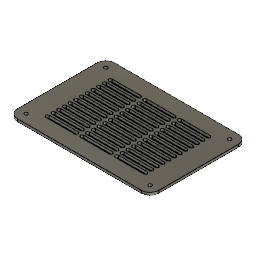
Maker Station v39 (Autodesk Fusion 360 design; units mm, degrees)
Autodesk Fusion 360 part; units mm, degrees
sketch "PiFaceplate" plane through (0, 0, 0) normal (0, 0, 1) x (1, 0, 0)
  line L0 (10, 0) -> (140, 0)
  line L1 (150, 10) -> (150, 100)
  line L2 (140, 110) -> (10, 110)
  line L3 (0, 100) -> (0, 10)
  line L4 (44.2438, 90.3301) -> (105.7438, 90.3301)
  line L5 (107.7438, 88.3301) -> (107.7438, 61.8301)
  line L6 (105.7438, 59.8301) -> (44.2438, 59.8301)
  line L7 (42.2438, 61.8301) -> (42.2438, 88.3301)
  line L8 (20, 40) -> (34.5, 40)
  line L9 (34.5, 40) -> (34.5, 32.75)
  line L10 (34.5, 32.75) -> (20, 32.75)
  line L11 (20, 32.75) -> (20, 40)
  line L12 (34.5, 32.75) -> (20, 32.75)
  line L13 (50, 40) -> (64.5, 40)
  line L14 (64.5, 40) -> (64.5, 32.75)
  line L15 (64.5, 32.75) -> (50, 32.75)
  line L16 (50, 32.75) -> (50, 40)
  line L17 (85.6117, 40) -> (100.1117, 40)
  line L18 (100.1117, 40) -> (100.1117, 32.75)
  line L19 (100.1117, 32.75) -> (85.6117, 32.75)
  line L20 (85.6117, 32.75) -> (85.6117, 40)
  line L21 (115.5147, 40) -> (130.0147, 40)
  line L22 (130.0147, 40) -> (130.0147, 32.75)
  line L23 (130.0147, 32.75) -> (115.5147, 32.75)
  line L24 (115.5147, 32.75) -> (115.5147, 40)
  arc A0 (44.2438, 90.3301) -> (42.2438, 88.3301) centre (44.2438, 88.3301) ccw
  arc A1 (42.2438, 61.8301) -> (44.2438, 59.8301) centre (44.2438, 61.8301) ccw
  arc A2 (107.7438, 88.3301) -> (105.7438, 90.3301) centre (105.7438, 88.3301) ccw
  arc A3 (105.7438, 59.8301) -> (107.7438, 61.8301) centre (105.7438, 61.8301) ccw
  arc A4 (150, 100) -> (140, 110) centre (140, 100) ccw
  arc A5 (140, 0) -> (150, 10) centre (140, 10) ccw
  arc A6 (10, 110) -> (0, 100) centre (10, 100) ccw
  arc A7 (0, 10) -> (10, 0) centre (10, 10) ccw
  line L25 (19.8132, 22.3848) -> (34.3132, 22.3848)
  line L26 (34.3132, 22.3848) -> (34.3132, 15.1348)
  line L27 (34.3132, 15.1348) -> (19.8132, 15.1348)
  line L28 (19.8132, 15.1348) -> (19.8132, 22.3848)
  line L29 (50, 22.3848) -> (64.5, 22.3848)
  line L30 (64.5, 22.3848) -> (64.5, 15.1348)
  line L31 (64.5, 15.1348) -> (50, 15.1348)
  line L32 (50, 15.1348) -> (50, 22.3848)
  line L33 (99.8132, 22.198) -> (85.3132, 22.198)
  line L34 (85.3132, 22.198) -> (85.3132, 14.948)
  line L35 (85.3132, 14.948) -> (99.8132, 14.948)
  line L36 (99.8132, 14.948) -> (99.8132, 22.198)
  line L37 (129.4396, 22.198) -> (114.9396, 22.198)
  line L38 (114.9396, 22.198) -> (114.9396, 14.948)
  line L39 (114.9396, 14.948) -> (129.4396, 14.948)
  line L40 (129.4396, 14.948) -> (129.4396, 22.198)
  circle A8 centre (10, 10) radius 2
  circle A9 centre (140, 10) radius 2
  circle A10 centre (140, 100) radius 2
  circle A11 centre (10, 100) radius 2
  dimension "d1" = 110
  dimension "d2" = 150
  dimension "d3" = 65.5
  dimension "d4" = 30.5
  dimension "d5" = 14.5
  dimension "d6" = 7.25
  dimension "d7" = 14.5
  dimension "d8" = 7.25
  dimension "d9" = 14.5
  dimension "d10" = 7.25
  dimension "d11" = 14.5
  dimension "d12" = 7.25
  dimension "d22" = 2
  dimension "d23" = 2
  dimension "d24" = 2
  dimension "d25" = 2
  dimension "d26" = 10
  dimension "d27" = 10
  dimension "d28" = 10
  dimension "d29" = 10
  dimension "d36" = 14.5
  dimension "d37" = 7.25
  dimension "d38" = 14.5
  dimension "d39" = 7.25
  dimension "d40" = 14.5
  dimension "d41" = 7.25
  dimension "d42" = 14.5
  dimension "d43" = 7.25
  dimension "d44" = 4
  dimension "d45" = 4
  dimension "d46" = 4
  dimension "d47" = 4
  measures "d22" radius of A0
  measures "d23" radius of A1
  measures "d24" radius of A2
  measures "d25" radius of A3
  measures "d26" radius of A4
  measures "d27" radius of A5
  measures "d28" radius of A6
  measures "d29" radius of A7
  measures "d36" distance of origin
  measures "d39" distance of origin
  measures "d41" distance of origin
  measures "d43" distance of origin
  measures "d44" diameter of A8
  measures "d45" diameter of A9
  measures "d46" diameter of A10
  measures "d47" diameter of A11
sketch "PiFaceplateUSB" plane through (0, 30, 0) normal (0, 1, 0) x (-1, 0, 0)
  line L0 (-15, -26) -> (-15, 0)
  line L1 (-135, 0) -> (-135, -26)
  line L2 (-135, -26) -> (-15, -26)
  line L3 (-132.2416, -2.0374) -> (-113.1416, -2.0374)
  line L4 (-113.1416, -2.0374) -> (-113.1416, -16.6374)
  line L5 (-113.1416, -16.6374) -> (-132.2416, -16.6374)
  line L6 (-132.2416, -16.6374) -> (-132.2416, -2.0374)
  line L7 (-102.384, -2.1628) -> (-83.284, -2.1628)
  line L8 (-83.284, -2.1628) -> (-83.284, -16.7628)
  line L9 (-83.284, -16.7628) -> (-102.384, -16.7628)
  line L10 (-102.384, -16.7628) -> (-102.384, -2.1628)
  line L11 (-66.6366, -2.2196) -> (-47.5366, -2.2196)
  line L12 (-47.5366, -2.2196) -> (-47.5366, -16.8196)
  line L13 (-47.5366, -16.8196) -> (-66.6366, -16.8196)
  line L14 (-66.6366, -16.8196) -> (-66.6366, -2.2196)
  line L15 (-37.0103, -2.4202) -> (-17.9103, -2.4202)
  line L16 (-17.9103, -2.4202) -> (-17.9103, -17.0202)
  line L17 (-17.9103, -17.0202) -> (-37.0103, -17.0202)
  line L18 (-37.0103, -17.0202) -> (-37.0103, -2.4202)
  line L19 (-135, 0) -> (-15, 0)
  line L20 (-15, 0) -> (-15, -21)
  line L21 (-20, -26) -> (-130, -26)
  line L22 (-135, -21) -> (-135, 0)
  arc A0 (-135, -21) -> (-130, -26) centre (-130, -21) ccw
  arc A1 (-20, -26) -> (-15, -21) centre (-20, -21) ccw
  line L23 (-15, 0) -> (-135, 0)
  dimension "d55" = 19.1
  dimension "d56" = 14.6
  dimension "d57" = 19.1
  dimension "d58" = 14.6
  dimension "d59" = 19.1
  dimension "d60" = 14.6
  dimension "d61" = 19.1
  dimension "d62" = 14.6
  dimension "d73" = 5
  dimension "d74" = 5
  measures "d73" radius of A0
  measures "d74" radius of A1
combine "Combine1" [no effect]
sketch "SwitchPlate" plane through (0, 0, 0) normal (0, 0, 1) x (1, 0, 0)
  line L0 (-102, 110) -> (-10.6, 110)
  line L1 (-0.6, 100) -> (-0.6, 10)
  line L2 (-10.6, 0) -> (-102, 0)
  line L3 (-112, 10) -> (-112, 100)
  arc A0 (-102, 110) -> (-112, 100) centre (-102, 100) ccw
  arc A1 (-0.6, 100) -> (-10.6, 110) centre (-10.6, 100) ccw
  arc A2 (-112, 10) -> (-102, 0) centre (-102, 10) ccw
  arc A3 (-10.6, 0) -> (-0.6, 10) centre (-10.6, 10) ccw
  circle A4 centre (-102, 100) radius 2
  circle A5 centre (-10.6, 100) radius 2
  circle A6 centre (-10.6, 10) radius 2
  circle A7 centre (-102, 10) radius 2
  circle A8 centre (-79.1, 91.075) radius 8
  circle A9 centre (-55.3, 91.075) radius 8
  circle A10 centre (-31.5, 91.075) radius 8
  circle A11 centre (-79.1, 73.225) radius 8
  circle A12 centre (-55.3, 73.225) radius 8
  circle A13 centre (-31.5, 73.225) radius 8
  circle A14 centre (-79.1, 55.375) radius 8
  circle A15 centre (-55.3, 55.375) radius 8
  circle A16 centre (-31.5, 55.375) radius 8
  circle A17 centre (-79.1, 37.525) radius 8
  circle A18 centre (-55.3, 37.525) radius 8
  circle A19 centre (-31.5, 37.525) radius 8
  circle A20 centre (-79.1, 19.675) radius 8
  circle A21 centre (-55.3, 19.675) radius 8
  circle A22 centre (-31.5, 19.675) radius 8
  dimension "d88" = 111.4
  dimension "d89" = 110
  dimension "d90" = 10
  dimension "d91" = 10
  dimension "d92" = 10
  dimension "d93" = 10
  dimension "d94" = 4
  dimension "d95" = 4
  dimension "d96" = 4
  dimension "d97" = 4
  dimension "d128" = 16
  dimension "d129" = 16
  dimension "d130" = 16
  dimension "d131" = 16
  dimension "d132" = 16
  dimension "d133" = 16
  dimension "d134" = 16
  dimension "d135" = 16
  dimension "d136" = 16
  dimension "d137" = 16
  dimension "d138" = 16
  dimension "d139" = 16
  dimension "d140" = 16
  dimension "d141" = 16
  dimension "d142" = 16
  measures "d90" radius of A0
  measures "d91" radius of A1
  measures "d92" radius of A2
  measures "d93" radius of A3
  measures "d94" diameter of A4
  measures "d95" diameter of A5
  measures "d96" diameter of A6
  measures "d97" diameter of A7
  measures "d128" diameter of A8
  measures "d129" diameter of A9
  measures "d130" diameter of A10
  measures "d131" diameter of A11
  measures "d132" diameter of A12
  measures "d133" diameter of A13
  measures "d134" diameter of A14
  measures "d135" diameter of A15
  measures "d136" diameter of A16
  measures "d137" diameter of A17
  measures "d138" diameter of A18
  measures "d139" diameter of A19
  measures "d140" diameter of A20
  measures "d141" diameter of A21
  measures "d142" diameter of A22
extrude "Extrude9" add sketch "SwitchPlate" along normal blind 3 makes body 1
combine "Combine2" [no effect]
combine "Combine3" [no effect]
combine "Combine4" [no effect]
sketch "SwitchBox" plane through (0, 0, 0) normal (0, 1, 0) x (1, 0, 0)
  line L0 (-10, 0) -> (-102, 0)
  line L1 (-112, 10) -> (-112, 98.329)
  line L2 (-102, 108.329) -> (-10, 108.329)
  line L3 (0, 98.329) -> (0, 10)
  arc A0 (-10, 0) -> (0, 10) centre (-10, 10) ccw
  arc A1 (-112, 10) -> (-102, 0) centre (-102, 10) ccw
  arc A2 (0, 98.329) -> (-10, 108.329) centre (-10, 98.329) ccw
  arc A3 (-102, 108.329) -> (-112, 98.329) centre (-102, 98.329) ccw
  line L4 (-102, 10) -> (-10, 98.329) construction
  line L5 (-10, 10) -> (-102, 98.329) construction
  line L6 (-87, 103.329) -> (-25, 103.329)
  line L7 (-15, 93.329) -> (-15, 15)
  line L8 (-25, 5) -> (-87, 5)
  line L9 (-97, 15) -> (-97, 93.329)
  line L10 (-97, 103.329) -> (-15, 5) construction
  line L11 (-15, 103.329) -> (-97, 5) construction
  arc A4 (-25, 5) -> (-15, 15) centre (-25, 15) ccw
  arc A5 (-97, 15) -> (-87, 5) centre (-87, 15) ccw
  arc A6 (-15, 93.329) -> (-25, 103.329) centre (-25, 93.329) ccw
  arc A7 (-87, 103.329) -> (-97, 93.329) centre (-87, 93.329) ccw
  dimension "d214" = 112
  dimension "d215" = 108.329
  dimension "d216" = 10
  dimension "d217" = 10
  dimension "d218" = 10
  dimension "d219" = 10
  dimension "d220" = 92
  dimension "d221" = 88.329
  dimension "d253" = 82
  dimension "d254" = 98.329
  dimension "d255" = 10
  dimension "d256" = 10
  dimension "d257" = 10
  dimension "d258" = 10
  measures "d216" radius of A0
  measures "d217" radius of A1
  measures "d218" radius of A2
  measures "d219" radius of A3
  measures "d220" distance of origin
  measures "d255" radius of A4
  measures "d256" radius of A5
  measures "d257" radius of A6
  measures "d258" radius of A7
sketch "SwitchBoxFloor" plane through (0, 0, 0) normal (0, 1, 0) x (-1, 0, 0)
  line L0 (87, -103.329) -> (25, -103.329)
  line L1 (15, -93.329) -> (15, -15)
  line L2 (25, -5) -> (87, -5)
  line L3 (97, -15) -> (97, -93.329)
  line L4 (97, -103.329) -> (15, -5) construction
  line L5 (15, -103.329) -> (97, -5) construction
  arc A0 (25, -5) -> (15, -15) centre (25, -15) ccw
  arc A1 (97, -15) -> (87, -5) centre (87, -15) ccw
  arc A2 (15, -93.329) -> (25, -103.329) centre (25, -93.329) ccw
  arc A3 (87, -103.329) -> (97, -93.329) centre (87, -93.329) ccw
  circle A4 centre (90.6, -45.7) radius 4
  circle A5 centre (21.5, -45.7) radius 4
  circle A6 centre (21.5, -95) radius 4
  circle A7 centre (90.6, -95) radius 4
  circle A8 centre (90.6, -45.7) radius 2
  circle A9 centre (21.5, -45.7) radius 2
  circle A10 centre (21.5, -95) radius 2
  circle A11 centre (90.6, -95) radius 2
  dimension "d259" = 82
  dimension "d260" = 98.329
  dimension "d261" = 10
  dimension "d262" = 10
  dimension "d263" = 10
  dimension "d264" = 10
  dimension "d422" = 69.1
  dimension "d423" = 49.3
  dimension "d424" = 8
  dimension "d425" = 8
  dimension "d426" = 8
  dimension "d427" = 8
  dimension "d428" = 4
  dimension "d429" = 4
  dimension "d430" = 4
  dimension "d431" = 4
  measures "d261" radius of A0
  measures "d262" radius of A1
  measures "d263" radius of A2
  measures "d264" radius of A3
  measures "d424" diameter of A4
  measures "d425" diameter of A5
  measures "d426" diameter of A6
  measures "d427" diameter of A7
  measures "d428" diameter of A8
  measures "d429" diameter of A9
  measures "d430" diameter of A10
  measures "d431" diameter of A11
extrude "Extrude18" add sketch "SwitchBox" along normal blind 40 separate body makes body 2
draft "Draft5" angle 10 neutral plane through (-10, 0, 0) pull (0, 0, 1) 1 faces at (-5, 40, -41.1097) on bodies 2
hole "Hole5" at (-102, 57.3381, -98.329) direction (0, -0.984808, -0.173648) diameter 4 depth 4 tip angle 180 bodies 2
hole "Hole6" at (-10, 57.3381, -98.329) direction (0, -0.984808, -0.173648) diameter 4 depth 4 tip angle 180 bodies 2
hole "Hole7" at (-102, 41.7633, -10) direction (0, -0.984808, -0.173648) diameter 4 depth 4 tip angle 180 bodies 2
hole "Hole8" at (-10, 41.7633, -10) direction (0, -0.984808, -0.173648) diameter 4 depth 4 tip angle 180 bodies 2
sketch "BoxJoin" plane through (0, 0, 0) normal (1, 0, 0) x (0, 1, 0)
  line L0 (0, 0) -> (40, 0)
  line L1 (40, 0) -> (40, -108.329)
  line L2 (40, -108.329) -> (0, -108.329)
  line L3 (0, -108.329) -> (0, 0)
  line L4 (40, 0) -> (0, -108.329)
  line L5 (40, -108.329) -> (0, 0)
  line L6 (12.5, -84.1645) -> (27.5, -84.1645)
  line L7 (27.5, -84.1645) -> (27.5, -24.1645)
  line L8 (27.5, -24.1645) -> (12.5, -24.1645)
  line L9 (12.5, -24.1645) -> (12.5, -84.1645)
  line L10 (12.5, -84.1645) -> (27.5, -24.1645) construction
  line L11 (27.5, -84.1645) -> (12.5, -24.1645) construction
  line L12 (20, -54.1645) -> (40, -54.1645)
  circle A0 centre (30, -54.1645) radius 2
  dimension "d281" = 108.329
  dimension "d282" = 40
  dimension "d283" = 15
  dimension "d284" = 60
  dimension "d285" = 4
  measures "d283" distance of L0.start
  measures "d285" diameter of A0
hole "Hole9" at (0, 27.5, -84.1645) at (0, 27.5, -24.1645) at (0, 12.5, -24.1645) at (0, 12.5, -84.1645) direction (-1, 0, 0) diameter 4 depth 30 tip angle 180 bodies 2
hole "Hole10" at (0, 30, -54.1645) direction (-1, 0, 0) diameter 30 depth 30 tip angle 180 bodies 2
extrude "Extrude19" add sketch "SwitchBoxFloor" along normal blind 3 contours L0 L1 L2 L3 A0 A1 A2 A3 | A4 | A5 | A6 | A7 | A8 | A9 | A10 | A11 bodies 2
sketch "PowerBox" plane through (0, 0, 0) normal (0, 1, 0) x (1, 0, 0)
  line L0 (48, 95.25) -> (152, 64.75) construction
  line L1 (152, 95.25) -> (48, 64.75) construction
  circle A0 centre (152, 64.75) radius 4
  circle A1 centre (48, 64.75) radius 4
  circle A2 centre (48, 95.25) radius 4
  circle A3 centre (152, 95.25) radius 4
  circle A4 centre (152, 64.75) radius 2
  circle A5 centre (152, 95.25) radius 2
  circle A6 centre (48, 64.75) radius 2
  circle A7 centre (48, 95.25) radius 2
  line L2 (100, 54.1645) -> (100, 5)
  line L3 (30, 108.329) -> (170, 108.329)
  line L4 (180, 98.329) -> (180, 10)
  line L5 (170, 0) -> (30, 0)
  line L6 (20, 10) -> (20, 98.329)
  arc A8 (170, 0) -> (180, 10) centre (170, 10) ccw
  arc A9 (20, 10) -> (30, 0) centre (30, 10) ccw
  arc A10 (180, 98.329) -> (170, 108.329) centre (170, 98.329) ccw
  arc A11 (30, 108.329) -> (20, 98.329) centre (30, 98.329) ccw
  line L7 (45, 103.329) -> (155, 103.329)
  line L8 (165, 93.329) -> (165, 15)
  line L9 (155, 5) -> (45, 5)
  line L10 (35, 15) -> (35, 93.329)
  line L11 (35, 103.329) -> (165, 5) construction
  line L12 (165, 103.329) -> (35, 5) construction
  arc A12 (155, 5) -> (165, 15) centre (155, 15) ccw
  arc A13 (35, 15) -> (45, 5) centre (45, 15) ccw
  arc A14 (165, 93.329) -> (155, 103.329) centre (155, 93.329) ccw
  arc A15 (45, 103.329) -> (35, 93.329) centre (45, 93.329) ccw
  dimension "d452" = 200
  dimension "d453" = 108.329
  dimension "d470" = 30.5
  dimension "d471" = 104
  dimension "d472" = 8
  dimension "d473" = 8
  dimension "d474" = 8
  dimension "d475" = 8
  dimension "d476" = 4
  dimension "d477" = 4
  dimension "d478" = 4
  dimension "d479" = 4
  dimension "d566" = 10
  dimension "d567" = 10
  dimension "d568" = 10
  dimension "d569" = 10
  dimension "d570" = 130
  dimension "d571" = 98.329
  dimension "d572" = 10
  dimension "d573" = 10
  dimension "d574" = 10
  dimension "d575" = 10
  measures "d472" diameter of A0
  measures "d473" diameter of A1
  measures "d474" diameter of A2
  measures "d475" diameter of A3
  measures "d476" diameter of A4
  measures "d477" diameter of A5
  measures "d478" diameter of A6
  measures "d479" diameter of A7
  measures "d566" radius of A8
  measures "d567" radius of A9
  measures "d568" radius of A10
  measures "d569" radius of A11
  measures "d571" distance of origin
  measures "d572" radius of A12
  measures "d573" radius of A13
  measures "d574" radius of A14
  measures "d575" radius of A15
extrude "Extrude56" add sketch "PowerBox" along normal blind 40 separate body contours L3 L4 L5 L6 A8 A9 A10 A11 makes body 3
extrude "Extrude57" add sketch "PowerBox" along normal blind 3 contours L7 L8 L9 L10 A12 A13 A14 A15 bodies 3
extrude "Extrude58" add sketch "PowerBox" along normal blind 8 contours A1 bodies 3
extrude "Extrude59" add sketch "PowerBox" along normal blind 3 contours A6 bodies 3
extrude "Extrude60" add sketch "PowerBox" along normal blind 3 separate body contours A7 makes body 4
extrude "Extrude61" add sketch "PowerBox" along normal blind 8 contours A2 bodies 3 4
extrude "Extrude62" add sketch "PowerBox" along normal blind 3 separate body contours A5 makes body 5
extrude "Extrude63" add sketch "PowerBox" along normal blind 8 contours A3 bodies 3 5
extrude "Extrude64" add sketch "PowerBox" along normal blind 3 separate body contours A4 makes body 6
extrude "Extrude65" add sketch "PowerBox" along normal blind 8 contours A0 bodies 3 6
draft "Draft9" angle 10 neutral plane through (170, 0, 0) pull (0, 0, 1) 1 faces at (175, 40, -41.1097) on bodies 3
move_body "Move7" bodies 3 to x (1, 0, 0) y (0, 1, 0) z (0, 0, 1) at (-20, 0, 0)
hole "Hole50" at (0, 27.5, -84.1645) at (0, 27.5, -24.1645) at (0, 12.5, -24.1645) at (0, 12.5, -84.1645) direction (1, 0, 0) diameter 4 depth 15 tip angle 180 bodies 3
hole "Hole51" at (0, 30.1179, -54.1346) direction (1, 0, 0) diameter 30 depth 15 tip angle 180 bodies 3
hole "Hole52" at (145, 8.5517, -80.2053) direction (1, 0, 0) diameter 9 depth 15 tip angle 180 bodies 3
move_body "Move8" bodies 3 to x (1, 0, 0) y (0, 1, 0) z (0, 0, 1) at (20, 0, 0)
hole "Hole53" at (170, 57.3381, -98.329) direction (0, -0.984808, -0.173648) diameter 4 depth 4 tip angle 180 bodies 3
hole "Hole54" at (170, 41.7633, -10) direction (0, -0.984808, -0.173648) diameter 4 depth 4 tip angle 180 bodies 3
hole "Hole55" at (30, 41.7633, -10) direction (0, -0.984808, -0.173648) diameter 4 depth 4 tip angle 180 bodies 3
hole "Hole56" at (30, 57.3381, -98.329) direction (0, -0.984808, -0.173648) diameter 4 depth 4 tip angle 180 bodies 3
hole "Hole57" at (35, 27.5, -84.1645) direction (-1, 0, 0) diameter 8 depth 4 tip angle 180 bodies 3
hole "Hole58" at (35, 12.5, -84.1645) direction (-1, 0, 0) diameter 8 depth 4 tip angle 180 bodies 3
hole "Hole59" at (35, 27.5, -24.1645) direction (-1, 0, 0) diameter 8 depth 4 tip angle 180 bodies 3
hole "Hole60" at (35, 12.5, -24.1645) direction (-1, 0, 0) diameter 8 depth 4 tip angle 180 bodies 3
sketch "PowerBoxFacePlateWithPiZero" plane through (0, 0, 0) normal (0, 0, 1) x (1, 0, 0)
  line L0 (20, 0) -> (160, 0)
  line L1 (170, 10) -> (170, 100)
  line L2 (160, 110) -> (20, 110)
  line L3 (10, 100) -> (10, 10)
  arc A0 (10, 10) -> (20, 0) centre (20, 10) ccw
  arc A1 (160, 0) -> (170, 10) centre (160, 10) ccw
  arc A2 (20, 110) -> (10, 100) centre (20, 100) ccw
  arc A3 (170, 100) -> (160, 110) centre (160, 100) ccw
  circle A4 centre (20, 10) radius 2
  circle A5 centre (160, 10) radius 2
  circle A6 centre (160, 100) radius 2
  circle A7 centre (20, 100) radius 2
  circle A8 centre (50, 80) radius 6
  circle A9 centre (130, 80) radius 6
  line L4 (120.9659, 48.9991) -> (59.4659, 48.9991)
  line L5 (57.4659, 46.9991) -> (57.4659, 20.4991)
  line L6 (59.4659, 18.4991) -> (120.9659, 18.4991)
  line L7 (122.9659, 20.4991) -> (122.9659, 46.9991)
  line L8 (122.9659, 48.9991) -> (57.4659, 18.4991) construction
  line L9 (57.4659, 48.9991) -> (122.9659, 18.4991) construction
  arc A10 (57.4659, 20.4991) -> (59.4659, 18.4991) centre (59.4659, 20.4991) ccw
  arc A11 (59.4659, 48.9991) -> (57.4659, 46.9991) centre (59.4659, 46.9991) ccw
  arc A12 (120.9659, 18.4991) -> (122.9659, 20.4991) centre (120.9659, 20.4991) ccw
  arc A13 (122.9659, 46.9991) -> (120.9659, 48.9991) centre (120.9659, 46.9991) ccw
  dimension "d631" = 110
  dimension "d632" = 160
  dimension "d633" = 10
  dimension "d634" = 10
  dimension "d635" = 10
  dimension "d636" = 10
  dimension "d637" = 4
  dimension "d638" = 4
  dimension "d639" = 4
  dimension "d640" = 4
  dimension "d641" = 12
  dimension "d642" = 12
  dimension "d643" = 30.5
  dimension "d644" = 65.5
  dimension "d645" = 2
  dimension "d646" = 2
  dimension "d647" = 2
  dimension "d648" = 2
  measures "d632" distance of origin
  measures "d633" radius of A0
  measures "d634" radius of A1
  measures "d635" radius of A2
  measures "d636" radius of A3
  measures "d637" diameter of A4
  measures "d638" diameter of A5
  measures "d639" diameter of A6
  measures "d640" diameter of A7
  measures "d641" diameter of A8
  measures "d642" diameter of A9
  measures "d643" distance of origin
  measures "d645" radius of A10
  measures "d646" radius of A11
  measures "d647" radius of A12
  measures "d648" radius of A13
extrude "Extrude66" add sketch "PowerBoxFacePlateWithPiZero" along normal blind 3 separate body makes body 7
sketch "SmallBoxUsbPlate" plane through (0, 0, 0) normal (0, 0, 1) x (1, 0, 0)
  line L0 (10, 0) -> (101.4, 0)
  line L1 (111.4, 10) -> (111.4, 100)
  line L2 (101.4, 110) -> (10, 110)
  line L3 (0, 100) -> (0, 10)
  arc A0 (0, 10) -> (10, 0) centre (10, 10) ccw
  arc A1 (101.4, 0) -> (111.4, 10) centre (101.4, 10) ccw
  arc A2 (111.4, 100) -> (101.4, 110) centre (101.4, 100) ccw
  arc A3 (10, 110) -> (0, 100) centre (10, 100) ccw
  line L4 (45.45, 22.125) -> (30.95, 22.125)
  line L5 (30.95, 22.125) -> (30.95, 14.875)
  line L6 (30.95, 14.875) -> (45.45, 14.875)
  line L7 (45.45, 14.875) -> (45.45, 22.125)
  line L8 (45.45, 22.125) -> (30.95, 14.875) construction
  line L9 (30.95, 22.125) -> (45.45, 14.875) construction
  line L10 (80.45, 22.125) -> (65.95, 22.125)
  line L11 (65.95, 22.125) -> (65.95, 14.875)
  line L12 (65.95, 14.875) -> (80.45, 14.875)
  line L13 (80.45, 14.875) -> (80.45, 22.125)
  line L14 (80.45, 22.125) -> (65.95, 14.875) construction
  line L15 (65.95, 22.125) -> (80.45, 14.875) construction
  line L16 (45.45, 40.125) -> (30.95, 40.125)
  line L17 (30.95, 40.125) -> (30.95, 32.875)
  line L18 (30.95, 32.875) -> (45.45, 32.875)
  line L19 (45.45, 32.875) -> (45.45, 40.125)
  line L20 (45.45, 40.125) -> (30.95, 32.875) construction
  line L21 (30.95, 40.125) -> (45.45, 32.875) construction
  line L22 (80.45, 40.125) -> (65.95, 40.125)
  line L23 (65.95, 40.125) -> (65.95, 32.875)
  line L24 (65.95, 32.875) -> (80.45, 32.875)
  line L25 (80.45, 32.875) -> (80.45, 40.125)
  line L26 (80.45, 40.125) -> (65.95, 32.875) construction
  line L27 (65.95, 40.125) -> (80.45, 32.875) construction
  line L28 (45.45, 77.125) -> (30.95, 77.125)
  line L29 (30.95, 77.125) -> (30.95, 69.875)
  line L30 (30.95, 69.875) -> (45.45, 69.875)
  line L31 (45.45, 69.875) -> (45.45, 77.125)
  line L32 (45.45, 77.125) -> (30.95, 69.875) construction
  line L33 (30.95, 77.125) -> (45.45, 69.875) construction
  line L34 (80.45, 77.125) -> (65.95, 77.125)
  line L35 (65.95, 77.125) -> (65.95, 69.875)
  line L36 (65.95, 69.875) -> (80.45, 69.875)
  line L37 (80.45, 69.875) -> (80.45, 77.125)
  line L38 (80.45, 77.125) -> (65.95, 69.875) construction
  line L39 (65.95, 77.125) -> (80.45, 69.875) construction
  line L40 (45.45, 95.125) -> (30.95, 95.125)
  line L41 (30.95, 95.125) -> (30.95, 87.875)
  line L42 (30.95, 87.875) -> (45.45, 87.875)
  line L43 (45.45, 87.875) -> (45.45, 95.125)
  line L44 (45.45, 95.125) -> (30.95, 87.875) construction
  line L45 (30.95, 95.125) -> (45.45, 87.875) construction
  line L46 (80.45, 95.125) -> (65.95, 95.125)
  line L47 (65.95, 95.125) -> (65.95, 87.875)
  line L48 (65.95, 87.875) -> (80.45, 87.875)
  line L49 (80.45, 87.875) -> (80.45, 95.125)
  line L50 (80.45, 95.125) -> (65.95, 87.875) construction
  line L51 (65.95, 95.125) -> (80.45, 87.875) construction
  line L52 (94.7, 83.5) -> (16.7, 83.5)
  line L53 (16.7, 83.5) -> (16.7, 81.5)
  line L54 (16.7, 81.5) -> (94.7, 81.5)
  line L55 (94.7, 81.5) -> (94.7, 83.5)
  line L56 (94.7, 83.5) -> (16.7, 81.5) construction
  line L57 (16.7, 83.5) -> (94.7, 81.5) construction
  line L58 (94.7, 28.5) -> (16.7, 28.5)
  line L59 (16.7, 28.5) -> (16.7, 26.5)
  line L60 (16.7, 26.5) -> (94.7, 26.5)
  line L61 (94.7, 26.5) -> (94.7, 28.5)
  line L62 (94.7, 28.5) -> (16.7, 26.5) construction
  line L63 (16.7, 28.5) -> (94.7, 26.5) construction
  circle A4 centre (10, 10) radius 2
  circle A5 centre (10, 100) radius 2
  circle A6 centre (101.4, 100) radius 2
  circle A7 centre (101.4, 10) radius 2
  dimension "d651" = 111.4
  dimension "d652" = 110
  dimension "d653" = 10
  dimension "d654" = 10
  dimension "d655" = 10
  dimension "d656" = 10
  dimension "d661" = 14.5
  dimension "d662" = 7.25
  dimension "d663" = 14.5
  dimension "d664" = 7.25
  dimension "d665" = 14.5
  dimension "d666" = 7.25
  dimension "d667" = 14.5
  dimension "d668" = 7.25
  dimension "d669" = 14.5
  dimension "d670" = 7.25
  dimension "d671" = 7.25
  dimension "d672" = 14.5
  dimension "d673" = 7.25
  dimension "d674" = 14.5
  dimension "d676" = 7.25
  dimension "d677" = 78
  dimension "d678" = 2
  dimension "d679" = 78
  dimension "d680" = 2
  dimension "d687" = 4
  dimension "d688" = 4
  dimension "d689" = 4
  dimension "d690" = 4
  measures "d653" radius of A0
  measures "d654" radius of A1
  measures "d655" radius of A2
  measures "d656" radius of A3
  measures "d662" distance of origin
  measures "d664" distance of origin
  measures "d677" distance of origin
  measures "d679" distance of origin
  measures "d687" diameter of A4
  measures "d688" diameter of A5
  measures "d689" diameter of A6
  measures "d690" diameter of A7
extrude "Extrude73" add sketch "SmallBoxUsbPlate" along normal blind 3 separate body makes body 8
sketch "SmallBoxUsbPlateUsbSupport" plane through (0, 0, 0) normal (0, 1, 0) x (1, 0, 0)
  line L0 (89.7, -24) -> (21.7, -24)
  line L1 (16.7, -19) -> (16.7, 0)
  line L2 (16.7, 0) -> (94.7, 0)
  line L3 (94.7, 0) -> (94.7, -19)
  arc A0 (89.7, -24) -> (94.7, -19) centre (89.7, -19) ccw
  arc A1 (16.7, -19) -> (21.7, -24) centre (21.7, -19) ccw
  circle A2 centre (28.2, -20.35) radius 1.65
  circle A3 centre (28.2, -5.65) radius 1.65
  circle A4 centre (48.2, -20.35) radius 1.65
  circle A5 centre (48.2, -5.65) radius 1.65
  circle A6 centre (63.2, -20.35) radius 1.65
  circle A7 centre (83.2, -20.35) radius 1.65
  circle A8 centre (83.2, -5.65) radius 1.65
  circle A9 centre (63.2, -5.65) radius 1.65
  dimension "d707" = 5
  dimension "d708" = 5
  dimension "d713" = 3.3
  dimension "d714" = 3.3
  dimension "d715" = 3.3
  dimension "d716" = 3.3
  dimension "d717" = 3.3
  dimension "d718" = 3.3
  dimension "d719" = 3.3
  dimension "d720" = 3.3
  measures "d707" radius of A0
  measures "d708" radius of A1
  measures "d713" diameter of A2
  measures "d714" diameter of A3
  measures "d715" diameter of A4
  measures "d716" diameter of A5
  measures "d717" diameter of A6
  measures "d718" diameter of A7
  measures "d719" diameter of A8
  measures "d720" diameter of A9
extrude "Extrude76" add sketch "SmallBoxUsbPlateUsbSupport" along normal blind 2 from surface at 26.5 bodies 8
extrude "Extrude77" add sketch "SmallBoxUsbPlateUsbSupport" along normal blind 2 from surface at 81.5 bodies 8
sketch "ComputeBox" plane through (0, 0, 0) normal (0, 1, 0) x (1, 0, 0)
  arc A0 (155, 5) -> (165, 15) centre (155, 15) ccw
  line L0 (165, 93.329) -> (165, 15)
  line L1 (121.0013, 97.1895) -> (63.0013, 48.1895) construction
  line L2 (155, 5) -> (45, 5)
  line L3 (165, 103.329) -> (35, 5) construction
  line L4 (35, 103.329) -> (165, 5) construction
  line L5 (180, 98.329) -> (180, 10)
  line L6 (35, 15) -> (35, 93.329)
  arc A1 (170, 0) -> (180, 10) centre (170, 10) ccw
  arc A2 (45, 103.329) -> (35, 93.329) centre (45, 93.329) ccw
  circle A3 centre (121.0013, 97.1895) radius 4
  circle A4 centre (63.0013, 48.1895) radius 4
  circle A5 centre (121.0013, 48.1895) radius 4
  arc A6 (20, 10) -> (30, 0) centre (30, 10) ccw
  arc A7 (30, 108.329) -> (20, 98.329) centre (30, 98.329) ccw
  circle A8 centre (63.0013, 97.1895) radius 2
  arc A9 (165, 93.329) -> (155, 103.329) centre (155, 93.329) ccw
  circle A10 centre (121.0013, 97.1895) radius 2
  arc A11 (35, 15) -> (45, 5) centre (45, 15) ccw
  circle A12 centre (121.0013, 48.1895) radius 2
  arc A13 (180, 98.329) -> (170, 108.329) centre (170, 98.329) ccw
  circle A14 centre (63.0013, 97.1895) radius 4
  circle A15 centre (63.0013, 48.1895) radius 2
  line L7 (20, 10) -> (20, 98.329)
  line L8 (63.0013, 97.1895) -> (121.0013, 48.1895) construction
  line L9 (45, 103.329) -> (155, 103.329)
  line L10 (30, 108.329) -> (170, 108.329)
  line L11 (170, 0) -> (30, 0)
  circle A16 centre (170, 10) radius 2
  circle A17 centre (170, 98.329) radius 2
  circle A18 centre (30, 10) radius 2
  circle A19 centre (30, 98.329) radius 2
  dimension "d727" = 200
  dimension "d728" = 108.329
  dimension "d731" = 8
  dimension "d732" = 8
  dimension "d733" = 8
  dimension "d734" = 8
  dimension "d735" = 4
  dimension "d736" = 4
  dimension "d737" = 4
  dimension "d738" = 4
  dimension "d739" = 10
  dimension "d740" = 10
  dimension "d741" = 10
  dimension "d742" = 10
  dimension "d743" = 130
  dimension "d744" = 98.329
  dimension "d745" = 10
  dimension "d746" = 10
  dimension "d747" = 10
  dimension "d748" = 10
  dimension "d805" = 4
  dimension "d806" = 4
  dimension "d807" = 4
  dimension "d808" = 4
  measures "d731" diameter of A5
  measures "d732" diameter of A4
  measures "d733" diameter of A14
  measures "d734" diameter of A3
  measures "d735" diameter of A12
  measures "d736" diameter of A10
  measures "d737" diameter of A15
  measures "d738" diameter of A8
  measures "d739" radius of A1
  measures "d740" radius of A6
  measures "d741" radius of A13
  measures "d742" radius of A7
  measures "d744" distance of origin
  measures "d745" radius of A0
  measures "d746" radius of A11
  measures "d747" radius of A9
  measures "d748" radius of A2
  measures "d805" diameter of A16
  measures "d806" diameter of A17
  measures "d807" diameter of A18
  measures "d808" diameter of A19
extrude "Extrude78" add sketch "ComputeBox" along normal blind 40 separate body contours L5 A1 A6 A7 A13 L7 L10 L11 | A16 | A17 | A18 | A19 makes body 9
extrude "Extrude79" add sketch "ComputeBox" along normal blind 3 contours A0 L0 L2 L6 A2 A9 A11 L9 bodies 9
extrude "Extrude80" add sketch "ComputeBox" along normal blind 3 separate body contours A15 makes body 10
extrude "Extrude81" add sketch "ComputeBox" along normal blind 8 contours A4 bodies 9 10
extrude "Extrude82" add sketch "ComputeBox" along normal blind 3 separate body contours A12 makes body 11
extrude "Extrude83" add sketch "ComputeBox" along normal blind 8 contours A5 bodies 9 11
extrude "Extrude84" add sketch "ComputeBox" along normal blind 3 separate body contours A10 makes body 12
extrude "Extrude85" add sketch "ComputeBox" along normal blind 8 contours A3 bodies 9 12
extrude "Extrude86" add sketch "ComputeBox" along normal blind 8 contours A14 bodies 9
extrude "Extrude87" add sketch "ComputeBox" along normal blind 3 contours A8 bodies 9
draft "Draft10" angle 10 neutral plane through (170, 0, 0) pull (0, 0, 1) 1 faces at (175, 40, -41.1097) on bodies 9
hole "Hole61" at (0, 30, -54.1645) direction (1, 0, 0) diameter 30 depth 200 tip angle 180 bodies 9
hole "Hole62" at (0, 27.5, -24.1645) at (0, 12.5, -24.1645) at (0, 27.5, -84.1645) at (0, 12.5, -84.1645) direction (1, 0, 0) diameter 4 depth 200 tip angle 180 bodies 9
hole "Hole63" at (165, 27.5, -24.1645) direction (1, 0, 0) diameter 8 depth 4 tip angle 180 bodies 9
hole "Hole64" at (165, 12.5, -24.1645) direction (1, 0, 0) diameter 8 depth 4 tip angle 180 bodies 9
hole "Hole65" at (165, 27.5, -84.1645) direction (1, 0, 0) diameter 8 depth 4 tip angle 180 bodies 9
hole "Hole66" at (165, 12.5, -84.1645) direction (1, 0, 0) diameter 8 depth 4 tip angle 180 bodies 9
hole "Hole67" at (35, 27.5, -84.1645) direction (-1, 0, 0) diameter 8 depth 4 tip angle 180 bodies 9
hole "Hole68" at (35, 12.5, -84.1645) direction (-1, 0, 0) diameter 8 depth 4 tip angle 180 bodies 9
hole "Hole69" at (35, 27.5, -24.1645) direction (-1, 0, 0) diameter 8 depth 4 tip angle 180 bodies 9
hole "Hole70" at (35, 12.5, -24.1645) direction (-1, 0, 0) diameter 8 depth 4 tip angle 180 bodies 9
hole "Hole71" at (170, 41.7633, -10) direction (0, -0.984808, -0.173648) diameter 4 depth 4 tip angle 180 bodies 9
hole "Hole72" at (170, 57.3381, -98.329) direction (0, -0.984808, -0.173648) diameter 4 depth 4 tip angle 180 bodies 9
hole "Hole73" at (30, 57.3381, -98.329) direction (0, -0.984808, -0.173648) diameter 4 depth 4 tip angle 180 bodies 9
hole "Hole74" at (30, 41.7633, -10) direction (0, -0.984808, -0.173648) diameter 4 depth 4 tip angle 180 bodies 9
sketch "Sketch33" plane through (0, 0, 0) normal (0, 0, 1) x (1, 0, 0)
  line L0 (10, 0) -> (150, 0)
  line L1 (160, 10) -> (160, 100)
  line L2 (150, 110) -> (10, 110)
  line L3 (0, 100) -> (0, 10)
  arc A0 (0, 10) -> (10, 0) centre (10, 10) ccw
  arc A1 (150, 0) -> (160, 10) centre (150, 10) ccw
  arc A2 (10, 110) -> (0, 100) centre (10, 100) ccw
  arc A3 (160, 100) -> (150, 110) centre (150, 100) ccw
  line L4 (10, 10) -> (150, 100)
  line L5 (150, 10) -> (10, 100)
  dimension "d821" = 160
  dimension "d822" = 110
  dimension "d823" = 10
  dimension "d824" = 10
  dimension "d825" = 10
  dimension "d826" = 10
  measures "d823" radius of A0
  measures "d824" radius of A1
  measures "d825" radius of A2
  measures "d826" radius of A3
extrude "Extrude88" add sketch "Sketch33" along normal blind 3 separate body makes body 13
sketch "Sketch34" plane through (0, 0, 0) normal (0, 0, -1) x (-1, 0, 0)
  arc A0 (-150, 110) -> (-160, 100) centre (-150, 100) ccw construction
  line L0 (-160, 100) -> (-160, 10) construction
  arc A1 (-160, 10) -> (-150, 0) centre (-150, 10) ccw construction
  line L1 (-150, 0) -> (-10, 0) construction
  arc A2 (-10, 0) -> (0, 10) centre (-10, 10) ccw construction
  line L2 (0, 10) -> (0, 100) construction
  arc A3 (0, 100) -> (-10, 110) centre (-10, 100) ccw construction
  line L3 (-10, 110) -> (-150, 110) construction
  line L4 (-102.8467, 21.455) -> (-135.46, 21.455)
  line L5 (-137.46, 19.455) -> (-137.46, 19.54)
  line L6 (-135.46, 17.54) -> (-102.8467, 17.54)
  line L7 (-100.8467, 19.54) -> (-100.8467, 19.455)
  arc A4 (-135.46, 21.455) -> (-137.46, 19.455) centre (-135.46, 19.455) ccw
  arc A5 (-137.46, 19.54) -> (-135.46, 17.54) centre (-135.46, 19.54) ccw
  arc A6 (-102.8467, 17.54) -> (-100.8467, 19.54) centre (-102.8467, 19.54) ccw
  arc A7 (-100.8467, 19.455) -> (-102.8467, 21.455) centre (-102.8467, 19.455) ccw
extrude "Extrude89" add sketch "Sketch34" against normal up to surface (3 mm away) separate body makes body 14
copy_body "CopyPasteBodies2" bodies 14 makes body 15
move_body "MoveBody1" bodies 15 to x (1, 0, 0) y (0, 1, 0) z (0, 0, 1) at (-39.1533, 0, 0)
copy_body "CopyPasteBodies3" bodies 14 makes body 16
move_body "MoveBody2" bodies 16 to x (1, 0, 0) y (0, 1, 0) z (0, 0, 1) at (-78.3067, 0, 0)
copy_body "CopyPasteBodies4" bodies 14 makes body 17
copy_body "CopyPasteBodies5" bodies 15 makes body 18
copy_body "CopyPasteBodies6" bodies 16 makes body 19
move_body "MoveBody3" bodies 17 18 19 to x (1, 0, 0) y (0, 1, 0) z (0, 0, 1) at (0, 6.455, 0)
copy_body "CopyPasteBodies7" bodies 14 makes body 20
copy_body "CopyPasteBodies8" bodies 15 makes body 21
copy_body "CopyPasteBodies9" bodies 16 makes body 22
move_body "MoveBody4" bodies 20 21 22 to x (1, 0, 0) y (0, 1, 0) z (0, 0, 1) at (0, 12.91, 0)
copy_body "CopyPasteBodies10" bodies 14 makes body 23
copy_body "CopyPasteBodies11" bodies 15 makes body 24
copy_body "CopyPasteBodies12" bodies 16 makes body 25
move_body "MoveBody5" bodies 23 24 25 to x (1, 0, 0) y (0, 1, 0) z (0, 0, 1) at (0, 19.365, 0)
copy_body "CopyPasteBodies13" bodies 14 makes body 26
copy_body "CopyPasteBodies14" bodies 15 makes body 27
copy_body "CopyPasteBodies15" bodies 16 makes body 28
move_body "MoveBody6" bodies 26 27 28 to x (1, 0, 0) y (0, 1, 0) z (0, 0, 1) at (0, 25.82, 0)
copy_body "CopyPasteBodies16" bodies 14 makes body 29
copy_body "CopyPasteBodies17" bodies 15 makes body 30
copy_body "CopyPasteBodies18" bodies 16 makes body 31
move_body "MoveBody7" bodies 29 30 31 to x (1, 0, 0) y (0, 1, 0) z (0, 0, 1) at (0, 32.275, 0)
copy_body "CopyPasteBodies19" bodies 14 makes body 32
copy_body "CopyPasteBodies20" bodies 15 makes body 33
copy_body "CopyPasteBodies21" bodies 16 makes body 34
move_body "MoveBody8" bodies 32 33 34 to x (1, 0, 0) y (0, 1, 0) z (0, 0, 1) at (0, 38.73, 0)
copy_body "CopyPasteBodies22" bodies 14 makes body 35
copy_body "CopyPasteBodies23" bodies 15 makes body 36
copy_body "CopyPasteBodies24" bodies 16 makes body 37
move_body "MoveBody9" bodies 35 36 37 to x (1, 0, 0) y (0, 1, 0) z (0, 0, 1) at (0, 45.185, 0)
copy_body "CopyPasteBodies25" bodies 14 makes body 38
copy_body "CopyPasteBodies26" bodies 15 makes body 39
copy_body "CopyPasteBodies27" bodies 16 makes body 40
move_body "MoveBody10" bodies 38 39 40 to x (1, 0, 0) y (0, 1, 0) z (0, 0, 1) at (0, 51.64, 0)
copy_body "CopyPasteBodies28" bodies 14 makes body 41
copy_body "CopyPasteBodies29" bodies 15 makes body 42
copy_body "CopyPasteBodies30" bodies 16 makes body 43
move_body "MoveBody11" bodies 41 42 43 to x (1, 0, 0) y (0, 1, 0) z (0, 0, 1) at (0, 58.095, 0)
copy_body "CopyPasteBodies31" bodies 14 makes body 44
copy_body "CopyPasteBodies32" bodies 15 makes body 45
copy_body "CopyPasteBodies33" bodies 16 makes body 46
move_body "MoveBody12" bodies 44 45 46 to x (1, 0, 0) y (0, 1, 0) z (0, 0, 1) at (0, 64.55, 0)
copy_body "CopyPasteBodies34" bodies 14 makes body 47
copy_body "CopyPasteBodies35" bodies 15 makes body 48
copy_body "CopyPasteBodies36" bodies 16 makes body 49
move_body "MoveBody13" bodies 47 48 49 to x (1, 0, 0) y (0, 1, 0) z (0, 0, 1) at (0, 71.005, 0)
combine "Combine14" operation cut target body 13 tool bodies 14 15 16 17 18 19 20 21 22 23 24 25 26 27 28 29 30 31 32 33 34 35 36 37 38 39 40 41 42 43 44 45 46 47 48 49
hole "Hole75" at (10, 100, 0) at (150, 100, 0) at (150, 10, 0) at (10, 10, 0) direction (0, 0, 1) diameter 4 depth 3 tip angle 180 bodies 13
extrude "Extrude70" [suppressed]
combine "Combine13" [suppressed]
extrude "Extrude71" [suppressed]
extrude "Extrude72" [suppressed]
extrude "Extrude37" [suppressed]
extrude "Extrude35" [suppressed]
extrude "Extrude38" [suppressed]
extrude "Extrude39" [suppressed]
extrude "Extrude40" [suppressed]
extrude "Extrude41" [suppressed]
extrude "Extrude42" [suppressed]
extrude "Extrude43" [suppressed]
extrude "Extrude44" [suppressed]
extrude "Extrude45" [suppressed]
combine "Combine12" [suppressed]
draft "Draft7" [suppressed]
hole "Hole36" [suppressed]
hole "Hole37" [suppressed]
hole "Hole38" [suppressed]
hole "Hole39" [suppressed]
hole "Hole40" [suppressed]
hole "Hole41" [suppressed]
hole "Hole42" [suppressed]
combine "Combine5" [suppressed]
combine "Combine7" [suppressed]
combine "Combine8" [suppressed]
combine "Combine9" [suppressed]
combine "Combine10" [suppressed]
extrude "Extrude28" [suppressed]
extrude "Extrude29" [suppressed]
hole "Hole20" [suppressed]
moveface "MoveFace8" [suppressed]
move_face "OffsetFaces1" [suppressed]
extrude "Extrude30" [suppressed]
hole "Hole21" [suppressed]
move_face "OffsetFaces2" [suppressed]
copy_body "CopyPasteBodies1" [suppressed]
move_body "Move6" [suppressed]
hole "Hole22" [suppressed]
hole "Hole23" [suppressed]
hole "Hole24" [suppressed]
hole "Hole25" [suppressed]
hole "Hole26" [suppressed]
hole "Hole27" [suppressed]
hole "Hole28" [suppressed]
hole "Hole29" [suppressed]
hole "Hole30" [suppressed]
hole "Hole31" [suppressed]
delete_face "DeleteFace2" [suppressed]
delete_face "DeleteFace3" [suppressed]
delete_face "DeleteFace4" [suppressed]
delete_face "DeleteFace5" [suppressed]
extrude "Extrude31" [suppressed]
extrude "Extrude32" [suppressed]
extrude "Extrude33" [suppressed]
extrude "Extrude34" [suppressed]
combine "Combine11" [suppressed]
hole "Hole32" [suppressed]
hole "Hole33" [suppressed]
hole "Hole34" [suppressed]
hole "Hole35" [suppressed]
extrude "Extrude36" [suppressed]
sketch "BoxJoins" plane through (0, 0, 0) normal (1, 0, 0) x (0, 1, 0)
  line L0 (0, 0) -> (25, 0)
  line L1 (25, 0) -> (25, -108.329)
  line L2 (25, -108.329) -> (0, -108.329)
  line L3 (0, -108.329) -> (0, 0)
  circle A0 centre (7.5, -25) radius 2
  circle A1 centre (17.5, -25) radius 2
  circle A2 centre (7.5, -83.329) radius 2
  circle A3 centre (17.5, -83.329) radius 2
  circle A4 centre (18.8333, -54.1645) radius 12.5
  dimension "d236" = 108.329
  dimension "d237" = 25
  dimension "d238" = 58.329
  dimension "d239" = 10
  dimension "d240" = 4
  dimension "d241" = 4
  dimension "d242" = 4
  dimension "d243" = 4
  dimension "d244" = 25
  measures "d240" diameter of A0
  measures "d241" diameter of A1
  measures "d242" diameter of A2
  measures "d243" diameter of A3
  measures "d244" diameter of A4
boxprimitive "BoxPrimitive2" [suppressed]
extrude "Extrude1" [suppressed]
hidden bodies 1 2 3 7 8 9
named bodies: "SwitchPlate", "SmallBoxLeft", "PiPlate", "SwitchBox", "SmallBoxDual", "PowerBox", "PowerBoxRight", "PowerBoxFacePlateWPiZero", "UsbPlateSmall", "SmallBoxUsbPlate", "ComputeBox", "LargeBoxVentFaceplate"
